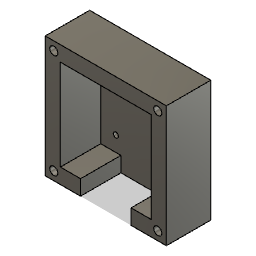
HQ Camera Case (main part) v7 (Autodesk Fusion 360 design; units mm, degrees)
Autodesk Fusion 360 part; units mm, degrees
sketch "Sketch1" plane through (0, 0, 0) normal (0, 0, 1) x (1, 0, 0)
  line L0 (-22.5, 22.5) -> (22.5, 22.5)
  line L1 (22.5, 22.5) -> (22.5, -22.5)
  line L2 (22.5, -22.5) -> (-22.5, -22.5)
  line L3 (-22.5, -22.5) -> (-22.5, 22.5)
  line L4 (-22.5, 22.5) -> (22.5, -22.5) construction
  line L5 (22.5, 22.5) -> (-22.5, -22.5) construction
  circle A0 centre (-15, 15) radius 1.25
  circle A1 centre (15, 15) radius 1.25
  circle A2 centre (15, -15) radius 1.25
  circle A3 centre (-15, -15) radius 1.25
  line L6 (-30, 30) -> (30, 30)
  line L7 (30, 30) -> (30, -30)
  line L8 (30, -30) -> (-30, -30)
  line L9 (-30, -30) -> (-30, 30)
  line L10 (-30, 30) -> (30, -30) construction
  line L11 (30, 30) -> (-30, -30) construction
  line L12 (-12.5, -22.5) -> (12.5, -22.5)
  line L13 (12.5, -22.5) -> (12.5, -30)
  line L14 (12.5, -30) -> (-12.5, -30)
  line L15 (-12.5, -30) -> (-12.5, -22.5)
  dimension "d1" = 45
  dimension "d2" = 45
  dimension "d3" = 2.5
  dimension "d4" = 2.5
  dimension "d5" = 2.5
  dimension "d6" = 2.5
  dimension "d7" = 7.5
  dimension "d9" = 7.5
  dimension "d10" = 7.5
  dimension "d11" = 7.5
  dimension "d12" = 60
  dimension "d13" = 60
  dimension "d14" = 7.5
  dimension "d15" = 10
  dimension "d16" = 10
  constraint horizontal L0
  constraint perpendicular L0 L1
  constraint parallel L0 L2
  constraint parallel L1 L3
  constraint coincident L4 origin
  constraint coincident L5 origin
  constraint coincident L4 A0.centre
  constraint coincident L5 A1.centre
  constraint coincident L4 A2.centre
  constraint coincident L5 A3.centre
  constraint horizontal L6
  constraint perpendicular L6 L7
  constraint parallel L6 L8
  constraint parallel L7 L9
  constraint coincident L10 origin
  constraint coincident L11 origin
  constraint horizontal L12
  constraint vertical L13
  constraint horizontal L14
  constraint vertical L15
  constraint coincident L2 L12.start
  measures "d1" distance of L1.end L2.end
  measures "d2" distance of L0.end L1.end
  measures "d3" diameter of A0
  measures "d4" diameter of A1
  measures "d5" diameter of A2
  measures "d6" diameter of A3
  measures "d7" distance of L3 A0.centre
  measures "d9" distance of L1 A1.centre
  measures "d10" distance of L3 A3.centre
  measures "d11" distance of L1 A2.centre
  measures "d12" distance of L7.end L8.end
  measures "d13" distance of L6.end L7.end
  measures "d14" distance of L12.start L14.end
  measures "d15" distance of L3 L15
  measures "d16" distance of L1 L13
extrude "Extrude1" add sketch "Sketch1" along normal blind 22 contours L0 L1 L2 L3 L6 L7 L8 L9 L13 L15
extrude "Extrude2" add sketch "Sketch1" along normal blind 2 contours L0 L1 L2 L3 L12
extrude "Extrude3" add sketch "Sketch1" along normal blind 2 contours L2 L8 L12 L13 L14 L15
sketch "Sketch2" plane through (0, 0, 22) normal (0, 0, 1) x (1, 0, 0)
  line L0 (-30, -30) -> (-12.5, -30)
  line L1 (-12.5, -30) -> (-12.5, -22.5)
  line L2 (-12.5, -22.5) -> (-22.5, -22.5)
  line L3 (-22.5, -22.5) -> (-22.5, 22.5)
  line L4 (-22.5, 22.5) -> (22.5, 22.5)
  line L5 (22.5, 22.5) -> (22.5, -22.5)
  line L6 (22.5, -22.5) -> (12.5, -22.5)
  line L7 (12.5, -22.5) -> (12.5, -30)
  line L8 (12.5, -30) -> (30, -30)
  line L9 (30, -30) -> (30, 30)
  line L10 (30, 30) -> (-30, 30)
  line L11 (-30, 30) -> (-30, -30)
  circle A0 centre (-25.75, 25.75) radius 2
  circle A1 centre (25.75, 25.75) radius 2
  circle A2 centre (-25.75, -25.75) radius 2
  circle A3 centre (25.75, -25.75) radius 2
  dimension "d23" = 4
  dimension "d24" = 4.25
  dimension "d25" = 4.25
  dimension "d26" = 4
  dimension "d27" = 4.25
  dimension "d28" = 4.25
  dimension "d29" = 4
  dimension "d30" = 4.25
  dimension "d31" = 4.25
  dimension "d32" = 4
  dimension "d33" = 4.25
  dimension "d34" = 4.25
  measures "d23" diameter of A0
  measures "d24" distance of L11 A0.centre
  measures "d25" distance of L10 A0.centre
  measures "d26" diameter of A1
  measures "d27" distance of L9 A1.centre
  measures "d28" distance of L10 A1.centre
  measures "d29" diameter of A2
  measures "d30" distance of L11 A2.centre
  measures "d31" distance of L0 A2.centre
  measures "d32" diameter of A3
  measures "d33" distance of L9 A3.centre
  measures "d34" distance of L8 A3.centre
extrude "Extrude4" cut sketch "Sketch2" against normal blind 4.72 contours A0 | A1 | A2 | A3
equation "d24 = holesfromcorner"
equation "d25 = holesfromcorner"
equation "d27 = holesfromcorner"
equation "d28 = holesfromcorner"
equation "d30 = holesfromcorner"
equation "d31 = holesfromcorner"
equation "d33 = holesfromcorner"
equation "d34 = holesfromcorner"
equation "holesfromcorner = 4.25 mm"
